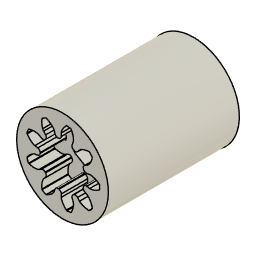
Motor Shaft (Autodesk Fusion 360 design; units mm, degrees)
description: Spur Gear; Module: 1.26; Num Teeth: 9; Pressure Angle: 20.0; Backlash: 0.00 mm
Autodesk Fusion 360 part; units mm, degrees
(part 1 of 2)
sketch "Sketch1" plane through (0, 0, 0) normal (0, 0, 1) x (1, 0, 0) in component "Spur Gear (9 teeth) (1)"
  circle A0 centre (0, 0) radius 4.1072
  circle A1 centre (0, 0) radius 2.5
extrude "Extrude1" add sketch "Sketch1" along normal blind 5 makes body 1 in component "Spur Gear (9 teeth) (1)"
sketch "Sketch2" plane through (0, 0, 0) normal (0, 0, 1) x (1, 0, 0) in component "Spur Gear (9 teeth) (1)"
  spline S0 degree 5 poles (5.2327, -1.0033) (5.2374, -1.0042) (5.2468, -1.0058) (5.2609, -1.0077) (5.2798, -1.0093) (5.3035, -1.0101) (5.3275, -1.0099) (5.3515, -1.0091) (5.3755, -1.008) (5.3996, -1.0067) (5.4238, -1.0051) (5.448, -1.0032) (5.4722, -1.0009) (5.4964, -0.9981) (5.5208, -0.9949) (5.5451, -0.9912) (5.5695, -0.9872) (5.5939, -0.9828) (5.6183, -0.9782) (5.6428, -0.9733) (5.6672, -0.9681) (5.6917, -0.9626) (5.7162, -0.9568) (5.7407, -0.9507) (5.7652, -0.9444) (5.7897, -0.9377) (5.8142, -0.9307) (5.8387, -0.9235) (5.8632, -0.916) (5.8877, -0.9083) (5.9123, -0.9003) (5.9368, -0.892) (5.9613, -0.8835) (5.9858, -0.8747) (6.0103, -0.8657) (6.0347, -0.8565) (6.0592, -0.847) (6.0837, -0.8372) (6.1081, -0.8272) (6.1325, -0.817) (6.1569, -0.8065) (6.1813, -0.7958) (6.2057, -0.7849) (6.23, -0.7738) (6.2543, -0.7624) (6.2786, -0.7508) (6.3029, -0.7389) (6.3271, -0.7269) (6.3513, -0.7146) (6.3755, -0.7021) (6.3997, -0.6894) (6.4238, -0.6765) (6.4479, -0.6633) (6.4719, -0.65) (6.4959, -0.6364) (6.5199, -0.6226) (6.5439, -0.6086) (6.5678, -0.5944) (6.5916, -0.58) (6.6154, -0.5653) (6.6392, -0.5505) (6.663, -0.5355) (6.6866, -0.5202) (6.7103, -0.5048) (6.7339, -0.4892) (6.7574, -0.4733) (6.7809, -0.4573) (6.8044, -0.441) (6.8278, -0.4246) (6.8511, -0.408) (6.8744, -0.3911) (6.893, -0.3775) (6.9069, -0.3672) (6.9162, -0.3603) (6.9208, -0.3568) knots 0 0 0 0 0 0 0.01428571 0.02857143 0.04285714 0.05714286 0.07142857 0.08571429 0.1 0.11428571 0.12857143 0.14285714 0.15714286 0.17142857 0.18571429 0.2 0.21428571 0.22857143 0.24285714 0.25714286 0.27142857 0.28571429 0.3 0.31428571 0.32857143 0.34285714 0.35714286 0.37142857 0.38571429 0.4 0.41428571 0.42857143 0.44285714 0.45714286 0.47142857 0.48571429 0.5 0.51428571 0.52857143 0.54285714 0.55714286 0.57142857 0.58571429 0.6 0.61428571 0.62857143 0.64285714 0.65714286 0.67142857 0.68571429 0.7 0.71428571 0.72857143 0.74285714 0.75714286 0.77142857 0.78571429 0.8 0.81428571 0.82857143 0.84285714 0.85714286 0.87142857 0.88571429 0.9 0.91428571 0.92857143 0.94285714 0.95714286 0.97142857 0.98571429 1 1 1 1 1 1
  spline S1 degree 5 poles (5.2327, 1.0033) (5.2374, 1.0042) (5.2468, 1.0058) (5.2609, 1.0077) (5.2798, 1.0093) (5.3035, 1.0101) (5.3275, 1.0099) (5.3515, 1.0091) (5.3755, 1.008) (5.3996, 1.0067) (5.4238, 1.0051) (5.448, 1.0032) (5.4722, 1.0009) (5.4964, 0.9981) (5.5208, 0.9949) (5.5451, 0.9912) (5.5695, 0.9872) (5.5939, 0.9828) (5.6183, 0.9782) (5.6428, 0.9733) (5.6672, 0.9681) (5.6917, 0.9626) (5.7162, 0.9568) (5.7407, 0.9507) (5.7652, 0.9444) (5.7897, 0.9377) (5.8142, 0.9307) (5.8387, 0.9235) (5.8632, 0.916) (5.8877, 0.9083) (5.9123, 0.9003) (5.9368, 0.892) (5.9613, 0.8835) (5.9858, 0.8747) (6.0103, 0.8657) (6.0347, 0.8565) (6.0592, 0.847) (6.0837, 0.8372) (6.1081, 0.8272) (6.1325, 0.817) (6.1569, 0.8065) (6.1813, 0.7958) (6.2057, 0.7849) (6.23, 0.7738) (6.2543, 0.7624) (6.2786, 0.7508) (6.3029, 0.7389) (6.3271, 0.7269) (6.3513, 0.7146) (6.3755, 0.7021) (6.3997, 0.6894) (6.4238, 0.6765) (6.4479, 0.6633) (6.4719, 0.65) (6.4959, 0.6364) (6.5199, 0.6226) (6.5439, 0.6086) (6.5678, 0.5944) (6.5916, 0.58) (6.6154, 0.5653) (6.6392, 0.5505) (6.663, 0.5355) (6.6866, 0.5202) (6.7103, 0.5048) (6.7339, 0.4892) (6.7574, 0.4733) (6.7809, 0.4573) (6.8044, 0.441) (6.8278, 0.4246) (6.8511, 0.408) (6.8744, 0.3911) (6.893, 0.3775) (6.9069, 0.3672) (6.9162, 0.3603) (6.9208, 0.3568) knots 0 0 0 0 0 0 0.01428571 0.02857143 0.04285714 0.05714286 0.07142857 0.08571429 0.1 0.11428571 0.12857143 0.14285714 0.15714286 0.17142857 0.18571429 0.2 0.21428571 0.22857143 0.24285714 0.25714286 0.27142857 0.28571429 0.3 0.31428571 0.32857143 0.34285714 0.35714286 0.37142857 0.38571429 0.4 0.41428571 0.42857143 0.44285714 0.45714286 0.47142857 0.48571429 0.5 0.51428571 0.52857143 0.54285714 0.55714286 0.57142857 0.58571429 0.6 0.61428571 0.62857143 0.64285714 0.65714286 0.67142857 0.68571429 0.7 0.71428571 0.72857143 0.74285714 0.75714286 0.77142857 0.78571429 0.8 0.81428571 0.82857143 0.84285714 0.85714286 0.87142857 0.88571429 0.9 0.91428571 0.92857143 0.94285714 0.95714286 0.97142857 0.98571429 1 1 1 1 1 1
  arc A0 (6.9208, -0.3568) -> (6.9208, 0.3568) centre (0, 0) ccw
  line L0 (4.0239, -0.7734) -> (5.2327, -1.0033)
  line L1 (4.0239, 0.7734) -> (5.2327, 1.0033)
  line L2 (4.0239, -0.7734) -> (4.0239, 0.7734)
  point P0 (5.3481, -1.0091)
  point P1 (5.4659, -1.0014)
  point P2 (5.5853, -0.9843)
  point P3 (5.7057, -0.9593)
  point P4 (5.8269, -0.9269)
  point P5 (5.9487, -0.8878)
  point P6 (6.0709, -0.8423)
  point P7 (6.1932, -0.7905)
  point P8 (6.3155, -0.7326)
  point P9 (6.4376, -0.6689)
  point P10 (6.5594, -0.5993)
  point P11 (6.6806, -0.5241)
  point P12 (6.8011, -0.4432)
  point P13 (5.3481, 1.0091)
  point P14 (5.4659, 1.0014)
  point P15 (5.5853, 0.9843)
  point P16 (5.7057, 0.9593)
  point P17 (5.8269, 0.9269)
  point P18 (5.9487, 0.8878)
  point P19 (6.0709, 0.8423)
  point P20 (6.1932, 0.7905)
  point P21 (6.3155, 0.7326)
  point P22 (6.4376, 0.6689)
  point P23 (6.5594, 0.5993)
  point P24 (6.6806, 0.5241)
  point P25 (6.8011, 0.4432)
extrude "Extrude2" add sketch "Sketch2" along normal blind 5 bodies 1 in component "Spur Gear (9 teeth) (1)"
fillet "Fillet1" radius 0.7 2 edges at (4.0334, -0.7752, 2.5) (4.0334, 0.7752, 2.5) on bodies 1 in component "Spur Gear (9 teeth) (1)"
pattern_circular "C-Pattern1" count 9 over 360 about axis through (0, 0, 0) along (0, 0, 1) of "Extrude2", "Fillet1" in component "Spur Gear (9 teeth) (1)"
sketch "Sketch3" plane through (0, 0, 0) normal (0, 0, 1) x (1, 0, 0) in component "Spur Gear (9 teeth) (1)"
  circle A0 centre (0, 0) radius 5.67 construction
move_body "Move1" bodies 1 to x (1, 0, 0) y (0, 0, -1) z (0, 1, 0) at (0, -13, 5) in component "Spur Gear (9 teeth) (1)"
sketch "Sketch5" plane through (0, -1, 0) normal (0, -1, 0) x (1, 0, 0)
  circle A0 centre (0, 0) radius 10
  circle A1 centre (0, 5) radius 2.5
  arc A2 (1.6934, 9.443) -> (2.0061, 8.584) centre (2.348, 9.1948) ccw
  line L0 (1.6934, 9.443) -> (1.8967, 9.979)
  spline S0 degree 5 poles (1.8967, 9.979) (1.8984, 9.9835) (1.9016, 9.9924) (1.906, 10.0059) (1.9108, 10.0243) (1.9157, 10.0476) (1.9196, 10.0712) (1.923, 10.0949) (1.9261, 10.1188) (1.929, 10.1428) (1.9316, 10.1668) (1.934, 10.191) (1.9359, 10.2152) (1.9374, 10.2396) (1.9385, 10.2641) (1.9391, 10.2887) (1.9393, 10.3135) (1.9393, 10.3383) (1.9389, 10.3631) (1.9383, 10.388) (1.9375, 10.413) (1.9363, 10.4381) (1.9349, 10.4632) (1.9332, 10.4884) (1.9311, 10.5136) (1.9288, 10.5389) (1.9262, 10.5642) (1.9233, 10.5896) (1.9202, 10.6151) (1.9169, 10.6406) (1.9132, 10.6661) (1.9094, 10.6917) (1.9052, 10.7173) (1.9009, 10.7429) (1.8962, 10.7686) (1.8914, 10.7943) (1.8863, 10.8201) (1.8809, 10.8459) (1.8753, 10.8717) (1.8695, 10.8975) (1.8634, 10.9233) (1.8571, 10.9492) (1.8506, 10.9751) (1.8438, 11.001) (1.8369, 11.0269) (1.8296, 11.0529) (1.8222, 11.0788) (1.8145, 11.1048) (1.8066, 11.1308) (1.7985, 11.1567) (1.7902, 11.1827) (1.7817, 11.2087) (1.7729, 11.2347) (1.7639, 11.2607) (1.7547, 11.2867) (1.7453, 11.3128) (1.7357, 11.3388) (1.7258, 11.3648) (1.7158, 11.3908) (1.7055, 11.4168) (1.695, 11.4428) (1.6844, 11.4687) (1.6735, 11.4947) (1.6624, 11.5207) (1.6511, 11.5466) (1.6395, 11.5726) (1.6278, 11.5985) (1.6159, 11.6244) (1.6038, 11.6503) (1.5914, 11.6762) (1.5789, 11.702) (1.5687, 11.7227) (1.561, 11.7382) (1.5558, 11.7485) (1.5532, 11.7537) knots 0 0 0 0 0 0 0.01428571 0.02857143 0.04285714 0.05714286 0.07142857 0.08571429 0.1 0.11428571 0.12857143 0.14285714 0.15714286 0.17142857 0.18571429 0.2 0.21428571 0.22857143 0.24285714 0.25714286 0.27142857 0.28571429 0.3 0.31428571 0.32857143 0.34285714 0.35714286 0.37142857 0.38571429 0.4 0.41428571 0.42857143 0.44285714 0.45714286 0.47142857 0.48571429 0.5 0.51428571 0.52857143 0.54285714 0.55714286 0.57142857 0.58571429 0.6 0.61428571 0.62857143 0.64285714 0.65714286 0.67142857 0.68571429 0.7 0.71428571 0.72857143 0.74285714 0.75714286 0.77142857 0.78571429 0.8 0.81428571 0.82857143 0.84285714 0.85714286 0.87142857 0.88571429 0.9 0.91428571 0.92857143 0.94285714 0.95714286 0.97142857 0.98571429 1 1 1 1 1 1
  arc A3 (1.5532, 11.7537) -> (0.8504, 11.8776) centre (0, 5) ccw
  spline S1 degree 5 poles (-0.0794, 10.3275) (-0.0795, 10.3322) (-0.0794, 10.3417) (-0.0789, 10.3559) (-0.0772, 10.3748) (-0.0738, 10.3984) (-0.0694, 10.4219) (-0.0645, 10.4454) (-0.0592, 10.4689) (-0.0537, 10.4924) (-0.048, 10.5159) (-0.0419, 10.5394) (-0.0355, 10.5629) (-0.0285, 10.5863) (-0.0211, 10.6097) (-0.0133, 10.633) (-0.0051, 10.6563) (0.0035, 10.6796) (0.0123, 10.7028) (0.0214, 10.726) (0.0307, 10.7492) (0.0404, 10.7724) (0.0503, 10.7955) (0.0606, 10.8185) (0.0711, 10.8416) (0.0819, 10.8645) (0.093, 10.8875) (0.1044, 10.9104) (0.1161, 10.9332) (0.1279, 10.956) (0.1401, 10.9788) (0.1525, 11.0015) (0.1651, 11.0241) (0.178, 11.0467) (0.1911, 11.0693) (0.2045, 11.0918) (0.2181, 11.1142) (0.2319, 11.1366) (0.246, 11.1589) (0.2603, 11.1812) (0.2749, 11.2034) (0.2896, 11.2256) (0.3046, 11.2477) (0.3198, 11.2697) (0.3353, 11.2917) (0.3509, 11.3136) (0.3668, 11.3354) (0.3829, 11.3572) (0.3991, 11.3789) (0.4157, 11.4006) (0.4324, 11.4222) (0.4493, 11.4437) (0.4664, 11.4651) (0.4838, 11.4865) (0.5013, 11.5078) (0.519, 11.529) (0.537, 11.5501) (0.5551, 11.5712) (0.5735, 11.5922) (0.592, 11.6131) (0.6107, 11.634) (0.6297, 11.6547) (0.6488, 11.6754) (0.6681, 11.696) (0.6876, 11.7165) (0.7073, 11.737) (0.7272, 11.7573) (0.7472, 11.7776) (0.7675, 11.7978) (0.7879, 11.8179) (0.8086, 11.8379) (0.8252, 11.8538) (0.8378, 11.8657) (0.8462, 11.8737) (0.8504, 11.8776) knots 0 0 0 0 0 0 0.01428571 0.02857143 0.04285714 0.05714286 0.07142857 0.08571429 0.1 0.11428571 0.12857143 0.14285714 0.15714286 0.17142857 0.18571429 0.2 0.21428571 0.22857143 0.24285714 0.25714286 0.27142857 0.28571429 0.3 0.31428571 0.32857143 0.34285714 0.35714286 0.37142857 0.38571429 0.4 0.41428571 0.42857143 0.44285714 0.45714286 0.47142857 0.48571429 0.5 0.51428571 0.52857143 0.54285714 0.55714286 0.57142857 0.58571429 0.6 0.61428571 0.62857143 0.64285714 0.65714286 0.67142857 0.68571429 0.7 0.71428571 0.72857143 0.74285714 0.75714286 0.77142857 0.78571429 0.8 0.81428571 0.82857143 0.84285714 0.85714286 0.87142857 0.88571429 0.9 0.91428571 0.92857143 0.94285714 0.95714286 0.97142857 0.98571429 1 1 1 1 1 1
  line L1 (-0.0794, 10.3275) -> (-0.0717, 9.7542)
  arc A4 (-0.6593, 9.0539) -> (-0.0717, 9.7542) centre (-0.7717, 9.7449) ccw
  arc A5 (-0.6593, 9.0539) -> (-0.767, 9.0349) centre (0, 5) ccw
  arc A6 (-1.5586, 9.4921) -> (-0.767, 9.0349) centre (-0.8977, 9.7226) ccw
  line L2 (-1.5586, 9.4921) -> (-1.7475, 10.0333)
  spline S2 degree 5 poles (-1.7475, 10.0333) (-1.749, 10.0378) (-1.7523, 10.0467) (-1.7577, 10.0599) (-1.7658, 10.0771) (-1.777, 10.098) (-1.7892, 10.1187) (-1.8018, 10.1391) (-1.8148, 10.1593) (-1.828, 10.1795) (-1.8415, 10.1997) (-1.8552, 10.2197) (-1.8693, 10.2395) (-1.8838, 10.2591) (-1.8988, 10.2786) (-1.9141, 10.2978) (-1.9298, 10.3169) (-1.9458, 10.3359) (-1.962, 10.3547) (-1.9785, 10.3734) (-1.9952, 10.392) (-2.0122, 10.4104) (-2.0294, 10.4288) (-2.047, 10.4469) (-2.0647, 10.465) (-2.0828, 10.4828) (-2.1011, 10.5006) (-2.1196, 10.5182) (-2.1383, 10.5357) (-2.1573, 10.5531) (-2.1765, 10.5703) (-2.1959, 10.5874) (-2.2155, 10.6044) (-2.2353, 10.6212) (-2.2554, 10.6379) (-2.2757, 10.6545) (-2.2961, 10.6709) (-2.3168, 10.6872) (-2.3377, 10.7034) (-2.3587, 10.7194) (-2.38, 10.7353) (-2.4014, 10.7511) (-2.4231, 10.7667) (-2.4449, 10.7822) (-2.4669, 10.7976) (-2.4891, 10.8128) (-2.5115, 10.8279) (-2.5341, 10.8429) (-2.5568, 10.8577) (-2.5797, 10.8724) (-2.6028, 10.887) (-2.6261, 10.9014) (-2.6495, 10.9157) (-2.6731, 10.9298) (-2.6969, 10.9438) (-2.7208, 10.9577) (-2.7449, 10.9714) (-2.7691, 10.985) (-2.7935, 10.9985) (-2.8181, 11.0118) (-2.8429, 11.025) (-2.8677, 11.038) (-2.8928, 11.0509) (-2.918, 11.0637) (-2.9433, 11.0763) (-2.9688, 11.0888) (-2.9945, 11.1011) (-3.0202, 11.1133) (-3.0462, 11.1253) (-3.0723, 11.1372) (-3.0985, 11.149) (-3.1196, 11.1583) (-3.1355, 11.1652) (-3.1461, 11.1697) (-3.1514, 11.172) knots 0 0 0 0 0 0 0.01428571 0.02857143 0.04285714 0.05714286 0.07142857 0.08571429 0.1 0.11428571 0.12857143 0.14285714 0.15714286 0.17142857 0.18571429 0.2 0.21428571 0.22857143 0.24285714 0.25714286 0.27142857 0.28571429 0.3 0.31428571 0.32857143 0.34285714 0.35714286 0.37142857 0.38571429 0.4 0.41428571 0.42857143 0.44285714 0.45714286 0.47142857 0.48571429 0.5 0.51428571 0.52857143 0.54285714 0.55714286 0.57142857 0.58571429 0.6 0.61428571 0.62857143 0.64285714 0.65714286 0.67142857 0.68571429 0.7 0.71428571 0.72857143 0.74285714 0.75714286 0.77142857 0.78571429 0.8 0.81428571 0.82857143 0.84285714 0.85714286 0.87142857 0.88571429 0.9 0.91428571 0.92857143 0.94285714 0.95714286 0.97142857 0.98571429 1 1 1 1 1 1
  arc A7 (-3.1514, 11.172) -> (-3.7694, 10.8152) centre (0, 5) ccw
  spline S3 degree 5 poles (-3.4853, 9.03) (-3.4884, 9.0336) (-3.4944, 9.0409) (-3.5031, 9.0522) (-3.514, 9.0677) (-3.5265, 9.088) (-3.5383, 9.1088) (-3.5496, 9.13) (-3.5607, 9.1514) (-3.5716, 9.1729) (-3.5823, 9.1946) (-3.5928, 9.2165) (-3.6029, 9.2386) (-3.6126, 9.261) (-3.622, 9.2837) (-3.631, 9.3066) (-3.6397, 9.3297) (-3.6481, 9.353) (-3.6563, 9.3765) (-3.6643, 9.4001) (-3.672, 9.4239) (-3.6795, 9.4478) (-3.6867, 9.4719) (-3.6937, 9.4962) (-3.7004, 9.5206) (-3.7069, 9.5452) (-3.7131, 9.5699) (-3.7191, 9.5947) (-3.7249, 9.6197) (-3.7305, 9.6448) (-3.7358, 9.67) (-3.7409, 9.6954) (-3.7458, 9.7209) (-3.7504, 9.7465) (-3.7549, 9.7722) (-3.7591, 9.798) (-3.7631, 9.8239) (-3.7669, 9.85) (-3.7704, 9.8762) (-3.7738, 9.9024) (-3.7769, 9.9288) (-3.7799, 9.9552) (-3.7826, 9.9818) (-3.7851, 10.0085) (-3.7874, 10.0352) (-3.7895, 10.0621) (-3.7914, 10.089) (-3.7931, 10.116) (-3.7945, 10.1431) (-3.7958, 10.1703) (-3.7969, 10.1976) (-3.7977, 10.2249) (-3.7984, 10.2524) (-3.7988, 10.2799) (-3.7991, 10.3075) (-3.7991, 10.3351) (-3.799, 10.3629) (-3.7986, 10.3907) (-3.7981, 10.4185) (-3.7973, 10.4465) (-3.7964, 10.4745) (-3.7952, 10.5026) (-3.7939, 10.5307) (-3.7923, 10.5589) (-3.7906, 10.5871) (-3.7886, 10.6155) (-3.7865, 10.6438) (-3.7841, 10.6723) (-3.7816, 10.7007) (-3.7789, 10.7293) (-3.7759, 10.7578) (-3.7734, 10.7808) (-3.7715, 10.798) (-3.7701, 10.8094) (-3.7694, 10.8152) knots 0 0 0 0 0 0 0.01428571 0.02857143 0.04285714 0.05714286 0.07142857 0.08571429 0.1 0.11428571 0.12857143 0.14285714 0.15714286 0.17142857 0.18571429 0.2 0.21428571 0.22857143 0.24285714 0.25714286 0.27142857 0.28571429 0.3 0.31428571 0.32857143 0.34285714 0.35714286 0.37142857 0.38571429 0.4 0.41428571 0.42857143 0.44285714 0.45714286 0.47142857 0.48571429 0.5 0.51428571 0.52857143 0.54285714 0.55714286 0.57142857 0.58571429 0.6 0.61428571 0.62857143 0.64285714 0.65714286 0.67142857 0.68571429 0.7 0.71428571 0.72857143 0.74285714 0.75714286 0.77142857 0.78571429 0.8 0.81428571 0.82857143 0.84285714 0.85714286 0.87142857 0.88571429 0.9 0.91428571 0.92857143 0.94285714 0.95714286 0.97142857 0.98571429 1 1 1 1 1 1
  line L3 (-3.4853, 9.03) -> (-3.1109, 8.5959)
  arc A8 (-3.1109, 7.6817) -> (-3.1109, 8.5959) centre (-3.6411, 8.1388) ccw
  arc A9 (-3.1109, 7.6817) -> (-3.1812, 7.5979) centre (0, 5) ccw
  arc A10 (-4.0814, 7.4392) -> (-3.1812, 7.5979) centre (-3.7233, 8.0407) ccw
  line L4 (-4.0814, 7.4392) -> (-4.574, 7.7325)
  spline S4 degree 5 poles (-4.574, 7.7325) (-4.5781, 7.7349) (-4.5863, 7.7396) (-4.5989, 7.7463) (-4.6161, 7.7543) (-4.6382, 7.7631) (-4.6608, 7.7711) (-4.6836, 7.7786) (-4.7066, 7.7857) (-4.7297, 7.7927) (-4.7529, 7.7995) (-4.7763, 7.806) (-4.7998, 7.8121) (-4.8236, 7.8178) (-4.8475, 7.8231) (-4.8717, 7.828) (-4.896, 7.8325) (-4.9204, 7.8368) (-4.9449, 7.8408) (-4.9696, 7.8445) (-4.9943, 7.848) (-5.0192, 7.8512) (-5.0442, 7.8542) (-5.0693, 7.8568) (-5.0945, 7.8592) (-5.1198, 7.8613) (-5.1452, 7.8632) (-5.1707, 7.8648) (-5.1963, 7.8661) (-5.222, 7.8672) (-5.2478, 7.8681) (-5.2737, 7.8687) (-5.2996, 7.8691) (-5.3256, 7.8692) (-5.3517, 7.8691) (-5.3779, 7.8688) (-5.4041, 7.8682) (-5.4304, 7.8674) (-5.4568, 7.8664) (-5.4832, 7.8652) (-5.5098, 7.8637) (-5.5363, 7.862) (-5.563, 7.86) (-5.5896, 7.8579) (-5.6164, 7.8555) (-5.6432, 7.8529) (-5.67, 7.8501) (-5.6969, 7.8471) (-5.7239, 7.8438) (-5.7509, 7.8403) (-5.7779, 7.8366) (-5.805, 7.8327) (-5.8322, 7.8286) (-5.8593, 7.8243) (-5.8865, 7.8197) (-5.9138, 7.815) (-5.9411, 7.81) (-5.9684, 7.8048) (-5.9957, 7.7995) (-6.0231, 7.7939) (-6.0505, 7.7881) (-6.078, 7.7821) (-6.1055, 7.7758) (-6.133, 7.7694) (-6.1605, 7.7628) (-6.188, 7.7559) (-6.2156, 7.7489) (-6.2432, 7.7417) (-6.2708, 7.7342) (-6.2984, 7.7266) (-6.3261, 7.7187) (-6.3482, 7.7123) (-6.3648, 7.7073) (-6.3759, 7.704) (-6.3814, 7.7024) knots 0 0 0 0 0 0 0.01428571 0.02857143 0.04285714 0.05714286 0.07142857 0.08571429 0.1 0.11428571 0.12857143 0.14285714 0.15714286 0.17142857 0.18571429 0.2 0.21428571 0.22857143 0.24285714 0.25714286 0.27142857 0.28571429 0.3 0.31428571 0.32857143 0.34285714 0.35714286 0.37142857 0.38571429 0.4 0.41428571 0.42857143 0.44285714 0.45714286 0.47142857 0.48571429 0.5 0.51428571 0.52857143 0.54285714 0.55714286 0.57142857 0.58571429 0.6 0.61428571 0.62857143 0.64285714 0.65714286 0.67142857 0.68571429 0.7 0.71428571 0.72857143 0.74285714 0.75714286 0.77142857 0.78571429 0.8 0.81428571 0.82857143 0.84285714 0.85714286 0.87142857 0.88571429 0.9 0.91428571 0.92857143 0.94285714 0.95714286 0.97142857 0.98571429 1 1 1 1 1 1
  arc A11 (-6.3814, 7.7024) -> (-6.6255, 7.0318) centre (0, 5) ccw
  spline S5 degree 5 poles (-5.2603, 5.8469) (-5.265, 5.8477) (-5.2743, 5.8494) (-5.2882, 5.8524) (-5.3066, 5.8573) (-5.3292, 5.8648) (-5.3516, 5.8731) (-5.3739, 5.8821) (-5.3961, 5.8913) (-5.4183, 5.9008) (-5.4404, 5.9106) (-5.4625, 5.9206) (-5.4845, 5.9311) (-5.5064, 5.942) (-5.5281, 5.9533) (-5.5497, 5.9651) (-5.5713, 5.9772) (-5.5927, 5.9897) (-5.6141, 6.0024) (-5.6353, 6.0154) (-5.6565, 6.0286) (-5.6777, 6.0421) (-5.6987, 6.0559) (-5.7196, 6.07) (-5.7405, 6.0844) (-5.7612, 6.0991) (-5.7819, 6.114) (-5.8024, 6.1292) (-5.8229, 6.1446) (-5.8433, 6.1602) (-5.8636, 6.1761) (-5.8838, 6.1923) (-5.9039, 6.2087) (-5.924, 6.2253) (-5.9439, 6.2421) (-5.9637, 6.2592) (-5.9835, 6.2765) (-6.0031, 6.294) (-6.0227, 6.3118) (-6.0421, 6.3297) (-6.0615, 6.3479) (-6.0807, 6.3663) (-6.0999, 6.3849) (-6.1189, 6.4037) (-6.1379, 6.4227) (-6.1567, 6.4419) (-6.1755, 6.4613) (-6.1942, 6.481) (-6.2127, 6.5008) (-6.2312, 6.5208) (-6.2495, 6.541) (-6.2678, 6.5614) (-6.2859, 6.582) (-6.3039, 6.6028) (-6.3218, 6.6237) (-6.3397, 6.6449) (-6.3574, 6.6662) (-6.375, 6.6878) (-6.3925, 6.7095) (-6.4098, 6.7314) (-6.4271, 6.7534) (-6.4443, 6.7757) (-6.4613, 6.7981) (-6.4783, 6.8207) (-6.4951, 6.8435) (-6.5118, 6.8664) (-6.5284, 6.8895) (-6.5449, 6.9128) (-6.5612, 6.9363) (-6.5775, 6.9599) (-6.5936, 6.9837) (-6.6064, 7.0028) (-6.616, 7.0173) (-6.6223, 7.0269) (-6.6255, 7.0318) knots 0 0 0 0 0 0 0.01428571 0.02857143 0.04285714 0.05714286 0.07142857 0.08571429 0.1 0.11428571 0.12857143 0.14285714 0.15714286 0.17142857 0.18571429 0.2 0.21428571 0.22857143 0.24285714 0.25714286 0.27142857 0.28571429 0.3 0.31428571 0.32857143 0.34285714 0.35714286 0.37142857 0.38571429 0.4 0.41428571 0.42857143 0.44285714 0.45714286 0.47142857 0.48571429 0.5 0.51428571 0.52857143 0.54285714 0.55714286 0.57142857 0.58571429 0.6 0.61428571 0.62857143 0.64285714 0.65714286 0.67142857 0.68571429 0.7 0.71428571 0.72857143 0.74285714 0.75714286 0.77142857 0.78571429 0.8 0.81428571 0.82857143 0.84285714 0.85714286 0.87142857 0.88571429 0.9 0.91428571 0.92857143 0.94285714 0.95714286 0.97142857 0.98571429 1 1 1 1 1 1
  line L5 (-5.2603, 5.8469) -> (-4.6945, 5.7549)
  arc A12 (-4.1068, 5.0547) -> (-4.6945, 5.7549) centre (-4.8068, 5.064) ccw
  arc A13 (-4.1068, 5.0547) -> (-4.1068, 4.9453) centre (0, 5) ccw
  arc A14 (-4.6945, 4.2451) -> (-4.1068, 4.9453) centre (-4.8068, 4.936) ccw
  line L6 (-4.6945, 4.2451) -> (-5.2603, 4.1531)
  spline S6 degree 5 poles (-5.2603, 4.1531) (-5.265, 4.1523) (-5.2743, 4.1506) (-5.2882, 4.1476) (-5.3066, 4.1427) (-5.3292, 4.1352) (-5.3516, 4.1269) (-5.3739, 4.1179) (-5.3961, 4.1087) (-5.4183, 4.0992) (-5.4404, 4.0894) (-5.4625, 4.0794) (-5.4845, 4.0689) (-5.5064, 4.058) (-5.5281, 4.0467) (-5.5497, 4.0349) (-5.5713, 4.0228) (-5.5927, 4.0103) (-5.6141, 3.9976) (-5.6353, 3.9846) (-5.6565, 3.9714) (-5.6777, 3.9579) (-5.6987, 3.9441) (-5.7196, 3.93) (-5.7405, 3.9156) (-5.7612, 3.9009) (-5.7819, 3.886) (-5.8024, 3.8708) (-5.8229, 3.8554) (-5.8433, 3.8398) (-5.8636, 3.8239) (-5.8838, 3.8077) (-5.9039, 3.7913) (-5.924, 3.7747) (-5.9439, 3.7579) (-5.9637, 3.7408) (-5.9835, 3.7235) (-6.0031, 3.706) (-6.0227, 3.6882) (-6.0421, 3.6703) (-6.0615, 3.6521) (-6.0807, 3.6337) (-6.0999, 3.6151) (-6.1189, 3.5963) (-6.1379, 3.5773) (-6.1567, 3.5581) (-6.1755, 3.5387) (-6.1942, 3.519) (-6.2127, 3.4992) (-6.2312, 3.4792) (-6.2495, 3.459) (-6.2678, 3.4386) (-6.2859, 3.418) (-6.3039, 3.3972) (-6.3218, 3.3763) (-6.3397, 3.3551) (-6.3574, 3.3338) (-6.375, 3.3122) (-6.3925, 3.2905) (-6.4098, 3.2686) (-6.4271, 3.2466) (-6.4443, 3.2243) (-6.4613, 3.2019) (-6.4783, 3.1793) (-6.4951, 3.1565) (-6.5118, 3.1336) (-6.5284, 3.1105) (-6.5449, 3.0872) (-6.5612, 3.0637) (-6.5775, 3.0401) (-6.5936, 3.0163) (-6.6064, 2.9972) (-6.616, 2.9827) (-6.6223, 2.9731) (-6.6255, 2.9682) knots 0 0 0 0 0 0 0.01428571 0.02857143 0.04285714 0.05714286 0.07142857 0.08571429 0.1 0.11428571 0.12857143 0.14285714 0.15714286 0.17142857 0.18571429 0.2 0.21428571 0.22857143 0.24285714 0.25714286 0.27142857 0.28571429 0.3 0.31428571 0.32857143 0.34285714 0.35714286 0.37142857 0.38571429 0.4 0.41428571 0.42857143 0.44285714 0.45714286 0.47142857 0.48571429 0.5 0.51428571 0.52857143 0.54285714 0.55714286 0.57142857 0.58571429 0.6 0.61428571 0.62857143 0.64285714 0.65714286 0.67142857 0.68571429 0.7 0.71428571 0.72857143 0.74285714 0.75714286 0.77142857 0.78571429 0.8 0.81428571 0.82857143 0.84285714 0.85714286 0.87142857 0.88571429 0.9 0.91428571 0.92857143 0.94285714 0.95714286 0.97142857 0.98571429 1 1 1 1 1 1
  arc A15 (-6.6255, 2.9682) -> (-6.3814, 2.2976) centre (0, 5) ccw
  spline S7 degree 5 poles (-4.574, 2.2675) (-4.5781, 2.2651) (-4.5863, 2.2604) (-4.5989, 2.2537) (-4.6161, 2.2457) (-4.6382, 2.2369) (-4.6608, 2.2289) (-4.6836, 2.2214) (-4.7066, 2.2143) (-4.7297, 2.2073) (-4.7529, 2.2005) (-4.7763, 2.194) (-4.7998, 2.1879) (-4.8236, 2.1822) (-4.8475, 2.1769) (-4.8717, 2.172) (-4.896, 2.1675) (-4.9204, 2.1632) (-4.9449, 2.1592) (-4.9696, 2.1555) (-4.9943, 2.152) (-5.0192, 2.1488) (-5.0442, 2.1458) (-5.0693, 2.1432) (-5.0945, 2.1408) (-5.1198, 2.1387) (-5.1452, 2.1368) (-5.1707, 2.1352) (-5.1963, 2.1339) (-5.222, 2.1328) (-5.2478, 2.1319) (-5.2737, 2.1313) (-5.2996, 2.1309) (-5.3256, 2.1308) (-5.3517, 2.1309) (-5.3779, 2.1312) (-5.4041, 2.1318) (-5.4304, 2.1326) (-5.4568, 2.1336) (-5.4832, 2.1348) (-5.5098, 2.1363) (-5.5363, 2.138) (-5.563, 2.14) (-5.5896, 2.1421) (-5.6164, 2.1445) (-5.6432, 2.1471) (-5.67, 2.1499) (-5.6969, 2.1529) (-5.7239, 2.1562) (-5.7509, 2.1597) (-5.7779, 2.1634) (-5.805, 2.1673) (-5.8322, 2.1714) (-5.8593, 2.1757) (-5.8865, 2.1803) (-5.9138, 2.185) (-5.9411, 2.19) (-5.9684, 2.1952) (-5.9957, 2.2005) (-6.0231, 2.2061) (-6.0505, 2.2119) (-6.078, 2.2179) (-6.1055, 2.2242) (-6.133, 2.2306) (-6.1605, 2.2372) (-6.188, 2.2441) (-6.2156, 2.2511) (-6.2432, 2.2583) (-6.2708, 2.2658) (-6.2984, 2.2734) (-6.3261, 2.2813) (-6.3482, 2.2877) (-6.3648, 2.2927) (-6.3759, 2.296) (-6.3814, 2.2976) knots 0 0 0 0 0 0 0.01428571 0.02857143 0.04285714 0.05714286 0.07142857 0.08571429 0.1 0.11428571 0.12857143 0.14285714 0.15714286 0.17142857 0.18571429 0.2 0.21428571 0.22857143 0.24285714 0.25714286 0.27142857 0.28571429 0.3 0.31428571 0.32857143 0.34285714 0.35714286 0.37142857 0.38571429 0.4 0.41428571 0.42857143 0.44285714 0.45714286 0.47142857 0.48571429 0.5 0.51428571 0.52857143 0.54285714 0.55714286 0.57142857 0.58571429 0.6 0.61428571 0.62857143 0.64285714 0.65714286 0.67142857 0.68571429 0.7 0.71428571 0.72857143 0.74285714 0.75714286 0.77142857 0.78571429 0.8 0.81428571 0.82857143 0.84285714 0.85714286 0.87142857 0.88571429 0.9 0.91428571 0.92857143 0.94285714 0.95714286 0.97142857 0.98571429 1 1 1 1 1 1
  line L7 (-4.574, 2.2675) -> (-4.0814, 2.5608)
  arc A16 (-3.1812, 2.4021) -> (-4.0814, 2.5608) centre (-3.7233, 1.9593) ccw
  arc A17 (-3.1812, 2.4021) -> (-3.1109, 2.3183) centre (0, 5) ccw
  arc A18 (-3.1109, 1.4041) -> (-3.1109, 2.3183) centre (-3.6411, 1.8612) ccw
  line L8 (-3.1109, 1.4041) -> (-3.4853, 0.97)
  spline S8 degree 5 poles (-3.4853, 0.97) (-3.4884, 0.9664) (-3.4944, 0.9591) (-3.5031, 0.9478) (-3.514, 0.9323) (-3.5265, 0.912) (-3.5383, 0.8912) (-3.5496, 0.87) (-3.5607, 0.8486) (-3.5716, 0.8271) (-3.5823, 0.8054) (-3.5928, 0.7835) (-3.6029, 0.7614) (-3.6126, 0.739) (-3.622, 0.7163) (-3.631, 0.6934) (-3.6397, 0.6703) (-3.6481, 0.647) (-3.6563, 0.6235) (-3.6643, 0.5999) (-3.672, 0.5761) (-3.6795, 0.5522) (-3.6867, 0.5281) (-3.6937, 0.5038) (-3.7004, 0.4794) (-3.7069, 0.4548) (-3.7131, 0.4301) (-3.7191, 0.4053) (-3.7249, 0.3803) (-3.7305, 0.3552) (-3.7358, 0.33) (-3.7409, 0.3046) (-3.7458, 0.2791) (-3.7504, 0.2535) (-3.7549, 0.2278) (-3.7591, 0.202) (-3.7631, 0.1761) (-3.7669, 0.15) (-3.7704, 0.1238) (-3.7738, 0.0976) (-3.7769, 0.0712) (-3.7799, 0.0448) (-3.7826, 0.0182) (-3.7851, -0.0085) (-3.7874, -0.0352) (-3.7895, -0.0621) (-3.7914, -0.089) (-3.7931, -0.116) (-3.7945, -0.1431) (-3.7958, -0.1703) (-3.7969, -0.1976) (-3.7977, -0.2249) (-3.7984, -0.2524) (-3.7988, -0.2799) (-3.7991, -0.3075) (-3.7991, -0.3351) (-3.799, -0.3629) (-3.7986, -0.3907) (-3.7981, -0.4185) (-3.7973, -0.4465) (-3.7964, -0.4745) (-3.7952, -0.5026) (-3.7939, -0.5307) (-3.7923, -0.5589) (-3.7906, -0.5871) (-3.7886, -0.6155) (-3.7865, -0.6438) (-3.7841, -0.6723) (-3.7816, -0.7007) (-3.7789, -0.7293) (-3.7759, -0.7578) (-3.7734, -0.7808) (-3.7715, -0.798) (-3.7701, -0.8094) (-3.7694, -0.8152) knots 0 0 0 0 0 0 0.01428571 0.02857143 0.04285714 0.05714286 0.07142857 0.08571429 0.1 0.11428571 0.12857143 0.14285714 0.15714286 0.17142857 0.18571429 0.2 0.21428571 0.22857143 0.24285714 0.25714286 0.27142857 0.28571429 0.3 0.31428571 0.32857143 0.34285714 0.35714286 0.37142857 0.38571429 0.4 0.41428571 0.42857143 0.44285714 0.45714286 0.47142857 0.48571429 0.5 0.51428571 0.52857143 0.54285714 0.55714286 0.57142857 0.58571429 0.6 0.61428571 0.62857143 0.64285714 0.65714286 0.67142857 0.68571429 0.7 0.71428571 0.72857143 0.74285714 0.75714286 0.77142857 0.78571429 0.8 0.81428571 0.82857143 0.84285714 0.85714286 0.87142857 0.88571429 0.9 0.91428571 0.92857143 0.94285714 0.95714286 0.97142857 0.98571429 1 1 1 1 1 1
  arc A19 (-3.7694, -0.8152) -> (-3.1514, -1.172) centre (0, 5) ccw
  spline S9 degree 5 poles (-1.7475, -0.0333) (-1.749, -0.0378) (-1.7523, -0.0467) (-1.7577, -0.0599) (-1.7658, -0.0771) (-1.777, -0.098) (-1.7892, -0.1187) (-1.8018, -0.1391) (-1.8148, -0.1593) (-1.828, -0.1795) (-1.8415, -0.1997) (-1.8552, -0.2197) (-1.8693, -0.2395) (-1.8838, -0.2591) (-1.8988, -0.2786) (-1.9141, -0.2978) (-1.9298, -0.3169) (-1.9458, -0.3359) (-1.962, -0.3547) (-1.9785, -0.3734) (-1.9952, -0.392) (-2.0122, -0.4104) (-2.0294, -0.4288) (-2.047, -0.4469) (-2.0647, -0.465) (-2.0828, -0.4828) (-2.1011, -0.5006) (-2.1196, -0.5182) (-2.1383, -0.5357) (-2.1573, -0.5531) (-2.1765, -0.5703) (-2.1959, -0.5874) (-2.2155, -0.6044) (-2.2353, -0.6212) (-2.2554, -0.6379) (-2.2757, -0.6545) (-2.2961, -0.6709) (-2.3168, -0.6872) (-2.3377, -0.7034) (-2.3587, -0.7194) (-2.38, -0.7353) (-2.4014, -0.7511) (-2.4231, -0.7667) (-2.4449, -0.7822) (-2.4669, -0.7976) (-2.4891, -0.8128) (-2.5115, -0.8279) (-2.5341, -0.8429) (-2.5568, -0.8577) (-2.5797, -0.8724) (-2.6028, -0.887) (-2.6261, -0.9014) (-2.6495, -0.9157) (-2.6731, -0.9298) (-2.6969, -0.9438) (-2.7208, -0.9577) (-2.7449, -0.9714) (-2.7691, -0.985) (-2.7935, -0.9985) (-2.8181, -1.0118) (-2.8429, -1.025) (-2.8677, -1.038) (-2.8928, -1.0509) (-2.918, -1.0637) (-2.9433, -1.0763) (-2.9688, -1.0888) (-2.9945, -1.1011) (-3.0202, -1.1133) (-3.0462, -1.1253) (-3.0723, -1.1372) (-3.0985, -1.149) (-3.1196, -1.1583) (-3.1355, -1.1652) (-3.1461, -1.1697) (-3.1514, -1.172) knots 0 0 0 0 0 0 0.01428571 0.02857143 0.04285714 0.05714286 0.07142857 0.08571429 0.1 0.11428571 0.12857143 0.14285714 0.15714286 0.17142857 0.18571429 0.2 0.21428571 0.22857143 0.24285714 0.25714286 0.27142857 0.28571429 0.3 0.31428571 0.32857143 0.34285714 0.35714286 0.37142857 0.38571429 0.4 0.41428571 0.42857143 0.44285714 0.45714286 0.47142857 0.48571429 0.5 0.51428571 0.52857143 0.54285714 0.55714286 0.57142857 0.58571429 0.6 0.61428571 0.62857143 0.64285714 0.65714286 0.67142857 0.68571429 0.7 0.71428571 0.72857143 0.74285714 0.75714286 0.77142857 0.78571429 0.8 0.81428571 0.82857143 0.84285714 0.85714286 0.87142857 0.88571429 0.9 0.91428571 0.92857143 0.94285714 0.95714286 0.97142857 0.98571429 1 1 1 1 1 1
  line L9 (-1.7475, -0.0333) -> (-1.5586, 0.5079)
  arc A20 (-0.767, 0.9651) -> (-1.5586, 0.5079) centre (-0.8977, 0.2774) ccw
  arc A21 (-0.767, 0.9651) -> (-0.6593, 0.9461) centre (0, 5) ccw
  arc A22 (-0.0717, 0.2458) -> (-0.6593, 0.9461) centre (-0.7717, 0.2551) ccw
  line L10 (-0.0717, 0.2458) -> (-0.0794, -0.3275)
  spline S10 degree 5 poles (-0.0794, -0.3275) (-0.0795, -0.3322) (-0.0794, -0.3417) (-0.0789, -0.3559) (-0.0772, -0.3748) (-0.0738, -0.3984) (-0.0694, -0.4219) (-0.0645, -0.4454) (-0.0592, -0.4689) (-0.0537, -0.4924) (-0.048, -0.5159) (-0.0419, -0.5394) (-0.0355, -0.5629) (-0.0285, -0.5863) (-0.0211, -0.6097) (-0.0133, -0.633) (-0.0051, -0.6563) (0.0035, -0.6796) (0.0123, -0.7028) (0.0214, -0.726) (0.0307, -0.7492) (0.0404, -0.7724) (0.0503, -0.7955) (0.0606, -0.8185) (0.0711, -0.8416) (0.0819, -0.8645) (0.093, -0.8875) (0.1044, -0.9104) (0.1161, -0.9332) (0.1279, -0.956) (0.1401, -0.9788) (0.1525, -1.0015) (0.1651, -1.0241) (0.178, -1.0467) (0.1911, -1.0693) (0.2045, -1.0918) (0.2181, -1.1142) (0.2319, -1.1366) (0.246, -1.1589) (0.2603, -1.1812) (0.2749, -1.2034) (0.2896, -1.2256) (0.3046, -1.2477) (0.3198, -1.2697) (0.3353, -1.2917) (0.3509, -1.3136) (0.3668, -1.3354) (0.3829, -1.3572) (0.3991, -1.3789) (0.4157, -1.4006) (0.4324, -1.4222) (0.4493, -1.4437) (0.4664, -1.4651) (0.4838, -1.4865) (0.5013, -1.5078) (0.519, -1.529) (0.537, -1.5501) (0.5551, -1.5712) (0.5735, -1.5922) (0.592, -1.6131) (0.6107, -1.634) (0.6297, -1.6547) (0.6488, -1.6754) (0.6681, -1.696) (0.6876, -1.7165) (0.7073, -1.737) (0.7272, -1.7573) (0.7472, -1.7776) (0.7675, -1.7978) (0.7879, -1.8179) (0.8086, -1.8379) (0.8252, -1.8538) (0.8378, -1.8657) (0.8462, -1.8737) (0.8504, -1.8776) knots 0 0 0 0 0 0 0.01428571 0.02857143 0.04285714 0.05714286 0.07142857 0.08571429 0.1 0.11428571 0.12857143 0.14285714 0.15714286 0.17142857 0.18571429 0.2 0.21428571 0.22857143 0.24285714 0.25714286 0.27142857 0.28571429 0.3 0.31428571 0.32857143 0.34285714 0.35714286 0.37142857 0.38571429 0.4 0.41428571 0.42857143 0.44285714 0.45714286 0.47142857 0.48571429 0.5 0.51428571 0.52857143 0.54285714 0.55714286 0.57142857 0.58571429 0.6 0.61428571 0.62857143 0.64285714 0.65714286 0.67142857 0.68571429 0.7 0.71428571 0.72857143 0.74285714 0.75714286 0.77142857 0.78571429 0.8 0.81428571 0.82857143 0.84285714 0.85714286 0.87142857 0.88571429 0.9 0.91428571 0.92857143 0.94285714 0.95714286 0.97142857 0.98571429 1 1 1 1 1 1
  arc A23 (0.8504, -1.8776) -> (1.5532, -1.7537) centre (0, 5) ccw
  spline S11 degree 5 poles (1.8967, 0.021) (1.8984, 0.0165) (1.9016, 0.0076) (1.906, -0.0059) (1.9108, -0.0243) (1.9157, -0.0476) (1.9196, -0.0712) (1.923, -0.0949) (1.9261, -0.1188) (1.929, -0.1428) (1.9316, -0.1668) (1.934, -0.191) (1.9359, -0.2152) (1.9374, -0.2396) (1.9385, -0.2641) (1.9391, -0.2887) (1.9393, -0.3135) (1.9393, -0.3383) (1.9389, -0.3631) (1.9383, -0.388) (1.9375, -0.413) (1.9363, -0.4381) (1.9349, -0.4632) (1.9332, -0.4884) (1.9311, -0.5136) (1.9288, -0.5389) (1.9262, -0.5642) (1.9233, -0.5896) (1.9202, -0.6151) (1.9169, -0.6406) (1.9132, -0.6661) (1.9094, -0.6917) (1.9052, -0.7173) (1.9009, -0.7429) (1.8962, -0.7686) (1.8914, -0.7943) (1.8863, -0.8201) (1.8809, -0.8459) (1.8753, -0.8717) (1.8695, -0.8975) (1.8634, -0.9233) (1.8571, -0.9492) (1.8506, -0.9751) (1.8438, -1.001) (1.8369, -1.0269) (1.8296, -1.0529) (1.8222, -1.0788) (1.8145, -1.1048) (1.8066, -1.1308) (1.7985, -1.1567) (1.7902, -1.1827) (1.7817, -1.2087) (1.7729, -1.2347) (1.7639, -1.2607) (1.7547, -1.2867) (1.7453, -1.3128) (1.7357, -1.3388) (1.7258, -1.3648) (1.7158, -1.3908) (1.7055, -1.4168) (1.695, -1.4428) (1.6844, -1.4687) (1.6735, -1.4947) (1.6624, -1.5207) (1.6511, -1.5466) (1.6395, -1.5726) (1.6278, -1.5985) (1.6159, -1.6244) (1.6038, -1.6503) (1.5914, -1.6762) (1.5789, -1.702) (1.5687, -1.7227) (1.561, -1.7382) (1.5558, -1.7485) (1.5532, -1.7537) knots 0 0 0 0 0 0 0.01428571 0.02857143 0.04285714 0.05714286 0.07142857 0.08571429 0.1 0.11428571 0.12857143 0.14285714 0.15714286 0.17142857 0.18571429 0.2 0.21428571 0.22857143 0.24285714 0.25714286 0.27142857 0.28571429 0.3 0.31428571 0.32857143 0.34285714 0.35714286 0.37142857 0.38571429 0.4 0.41428571 0.42857143 0.44285714 0.45714286 0.47142857 0.48571429 0.5 0.51428571 0.52857143 0.54285714 0.55714286 0.57142857 0.58571429 0.6 0.61428571 0.62857143 0.64285714 0.65714286 0.67142857 0.68571429 0.7 0.71428571 0.72857143 0.74285714 0.75714286 0.77142857 0.78571429 0.8 0.81428571 0.82857143 0.84285714 0.85714286 0.87142857 0.88571429 0.9 0.91428571 0.92857143 0.94285714 0.95714286 0.97142857 0.98571429 1 1 1 1 1 1
  line L11 (1.8967, 0.021) -> (1.6934, 0.557)
  arc A24 (2.0061, 1.416) -> (1.6934, 0.557) centre (2.348, 0.8052) ccw
  arc A25 (2.0061, 1.416) -> (2.1008, 1.4707) centre (0, 5) ccw
  arc A26 (3.001, 1.3119) -> (2.1008, 1.4707) centre (2.4588, 0.8692) ccw
  line L12 (3.001, 1.3119) -> (3.3636, 0.8679)
  spline S12 degree 5 poles (3.3636, 0.8679) (3.3666, 0.8642) (3.3727, 0.857) (3.3823, 0.8464) (3.3957, 0.833) (3.4135, 0.8172) (3.4319, 0.802) (3.4508, 0.7871) (3.47, 0.7725) (3.4893, 0.758) (3.5088, 0.7437) (3.5285, 0.7296) (3.5486, 0.7158) (3.5689, 0.7023) (3.5896, 0.6892) (3.6106, 0.6763) (3.6319, 0.6638) (3.6534, 0.6514) (3.6751, 0.6393) (3.697, 0.6273) (3.7191, 0.6156) (3.7413, 0.6041) (3.7638, 0.5927) (3.7865, 0.5817) (3.8094, 0.5708) (3.8324, 0.5602) (3.8557, 0.5497) (3.8791, 0.5395) (3.9027, 0.5295) (3.9265, 0.5197) (3.9504, 0.51) (3.9745, 0.5006) (3.9987, 0.4914) (4.0231, 0.4823) (4.0476, 0.4735) (4.0724, 0.4649) (4.0972, 0.4564) (4.1222, 0.4482) (4.1473, 0.4401) (4.1726, 0.4322) (4.198, 0.4246) (4.2236, 0.4171) (4.2493, 0.4098) (4.2751, 0.4027) (4.301, 0.3958) (4.3271, 0.3891) (4.3533, 0.3825) (4.3796, 0.3762) (4.4061, 0.37) (4.4326, 0.364) (4.4593, 0.3583) (4.4861, 0.3527) (4.513, 0.3473) (4.54, 0.342) (4.5671, 0.337) (4.5944, 0.3321) (4.6217, 0.3275) (4.6491, 0.323) (4.6767, 0.3187) (4.7043, 0.3146) (4.7321, 0.3107) (4.7599, 0.3069) (4.7879, 0.3034) (4.8159, 0.3) (4.844, 0.2968) (4.8723, 0.2938) (4.9006, 0.291) (4.929, 0.2884) (4.9575, 0.2859) (4.986, 0.2837) (5.0147, 0.2816) (5.0377, 0.2801) (5.055, 0.279) (5.0665, 0.2784) (5.0723, 0.2781) knots 0 0 0 0 0 0 0.01428571 0.02857143 0.04285714 0.05714286 0.07142857 0.08571429 0.1 0.11428571 0.12857143 0.14285714 0.15714286 0.17142857 0.18571429 0.2 0.21428571 0.22857143 0.24285714 0.25714286 0.27142857 0.28571429 0.3 0.31428571 0.32857143 0.34285714 0.35714286 0.37142857 0.38571429 0.4 0.41428571 0.42857143 0.44285714 0.45714286 0.47142857 0.48571429 0.5 0.51428571 0.52857143 0.54285714 0.55714286 0.57142857 0.58571429 0.6 0.61428571 0.62857143 0.64285714 0.65714286 0.67142857 0.68571429 0.7 0.71428571 0.72857143 0.74285714 0.75714286 0.77142857 0.78571429 0.8 0.81428571 0.82857143 0.84285714 0.85714286 0.87142857 0.88571429 0.9 0.91428571 0.92857143 0.94285714 0.95714286 0.97142857 0.98571429 1 1 1 1 1 1
  arc A27 (5.0723, 0.2781) -> (5.531, 0.8247) centre (0, 5) ccw
  spline S13 degree 5 poles (4.6534, 2.405) (4.6576, 2.4027) (4.6658, 2.3979) (4.6778, 2.3904) (4.6933, 2.3794) (4.712, 2.3647) (4.7302, 2.3492) (4.7481, 2.3332) (4.7658, 2.3168) (4.7834, 2.3003) (4.8009, 2.2836) (4.8182, 2.2666) (4.8353, 2.2493) (4.8521, 2.2316) (4.8687, 2.2135) (4.885, 2.195) (4.901, 2.1762) (4.9169, 2.1572) (4.9327, 2.1379) (4.9482, 2.1185) (4.9636, 2.0988) (4.9788, 2.0788) (4.9939, 2.0587) (5.0087, 2.0383) (5.0234, 2.0176) (5.0379, 1.9968) (5.0522, 1.9757) (5.0663, 1.9544) (5.0803, 1.9329) (5.0941, 1.9112) (5.1077, 1.8893) (5.1212, 1.8672) (5.1345, 1.845) (5.1476, 1.8225) (5.1606, 1.7999) (5.1734, 1.777) (5.186, 1.754) (5.1985, 1.7308) (5.2108, 1.7075) (5.2229, 1.6839) (5.2349, 1.6603) (5.2467, 1.6364) (5.2583, 1.6124) (5.2698, 1.5882) (5.2811, 1.5638) (5.2923, 1.5393) (5.3033, 1.5146) (5.3141, 1.4898) (5.3247, 1.4649) (5.3352, 1.4397) (5.3456, 1.4145) (5.3557, 1.3891) (5.3657, 1.3635) (5.3756, 1.3378) (5.3852, 1.312) (5.3947, 1.286) (5.4041, 1.2599) (5.4133, 1.2336) (5.4223, 1.2073) (5.4311, 1.1808) (5.4398, 1.1541) (5.4483, 1.1273) (5.4567, 1.1004) (5.4649, 1.0734) (5.4729, 1.0463) (5.4807, 1.019) (5.4884, 0.9916) (5.4959, 0.9641) (5.5033, 0.9364) (5.5105, 0.9087) (5.5175, 0.8808) (5.523, 0.8585) (5.527, 0.8416) (5.5297, 0.8304) (5.531, 0.8247) knots 0 0 0 0 0 0 0.01428571 0.02857143 0.04285714 0.05714286 0.07142857 0.08571429 0.1 0.11428571 0.12857143 0.14285714 0.15714286 0.17142857 0.18571429 0.2 0.21428571 0.22857143 0.24285714 0.25714286 0.27142857 0.28571429 0.3 0.31428571 0.32857143 0.34285714 0.35714286 0.37142857 0.38571429 0.4 0.41428571 0.42857143 0.44285714 0.45714286 0.47142857 0.48571429 0.5 0.51428571 0.52857143 0.54285714 0.55714286 0.57142857 0.58571429 0.6 0.61428571 0.62857143 0.64285714 0.65714286 0.67142857 0.68571429 0.7 0.71428571 0.72857143 0.74285714 0.75714286 0.77142857 0.78571429 0.8 0.81428571 0.82857143 0.84285714 0.85714286 0.87142857 0.88571429 0.9 0.91428571 0.92857143 0.94285714 0.95714286 0.97142857 0.98571429 1 1 1 1 1 1
  line L13 (4.6534, 2.405) -> (4.1532, 2.685)
  arc A28 (3.8405, 3.544) -> (4.1532, 2.685) centre (4.495, 3.2958) ccw
  arc A29 (3.8405, 3.544) -> (3.8779, 3.6468) centre (0, 5) ccw
  arc A30 (4.6696, 4.1038) -> (3.8779, 3.6468) centre (4.5388, 3.4161) ccw
  line L14 (4.6696, 4.1038) -> (5.2327, 3.9967)
  spline S14 degree 5 poles (5.2327, 3.9967) (5.2374, 3.9958) (5.2468, 3.9942) (5.2609, 3.9923) (5.2798, 3.9907) (5.3035, 3.9899) (5.3275, 3.9901) (5.3515, 3.9909) (5.3755, 3.992) (5.3996, 3.9933) (5.4238, 3.9949) (5.448, 3.9968) (5.4722, 3.9991) (5.4964, 4.0019) (5.5208, 4.0051) (5.5451, 4.0088) (5.5695, 4.0128) (5.5939, 4.0172) (5.6183, 4.0218) (5.6428, 4.0267) (5.6672, 4.0319) (5.6917, 4.0374) (5.7162, 4.0432) (5.7407, 4.0493) (5.7652, 4.0556) (5.7897, 4.0623) (5.8142, 4.0693) (5.8387, 4.0765) (5.8632, 4.084) (5.8877, 4.0917) (5.9123, 4.0997) (5.9368, 4.108) (5.9613, 4.1165) (5.9858, 4.1253) (6.0103, 4.1343) (6.0347, 4.1435) (6.0592, 4.153) (6.0837, 4.1628) (6.1081, 4.1728) (6.1325, 4.183) (6.1569, 4.1935) (6.1813, 4.2042) (6.2057, 4.2151) (6.23, 4.2262) (6.2543, 4.2376) (6.2786, 4.2492) (6.3029, 4.2611) (6.3271, 4.2731) (6.3513, 4.2854) (6.3755, 4.2979) (6.3997, 4.3106) (6.4238, 4.3235) (6.4479, 4.3367) (6.4719, 4.35) (6.4959, 4.3636) (6.5199, 4.3774) (6.5439, 4.3914) (6.5678, 4.4056) (6.5916, 4.42) (6.6154, 4.4347) (6.6392, 4.4495) (6.663, 4.4645) (6.6866, 4.4798) (6.7103, 4.4952) (6.7339, 4.5108) (6.7574, 4.5267) (6.7809, 4.5427) (6.8044, 4.559) (6.8278, 4.5754) (6.8511, 4.592) (6.8744, 4.6089) (6.893, 4.6225) (6.9069, 4.6328) (6.9162, 4.6397) (6.9208, 4.6432) knots 0 0 0 0 0 0 0.01428571 0.02857143 0.04285714 0.05714286 0.07142857 0.08571429 0.1 0.11428571 0.12857143 0.14285714 0.15714286 0.17142857 0.18571429 0.2 0.21428571 0.22857143 0.24285714 0.25714286 0.27142857 0.28571429 0.3 0.31428571 0.32857143 0.34285714 0.35714286 0.37142857 0.38571429 0.4 0.41428571 0.42857143 0.44285714 0.45714286 0.47142857 0.48571429 0.5 0.51428571 0.52857143 0.54285714 0.55714286 0.57142857 0.58571429 0.6 0.61428571 0.62857143 0.64285714 0.65714286 0.67142857 0.68571429 0.7 0.71428571 0.72857143 0.74285714 0.75714286 0.77142857 0.78571429 0.8 0.81428571 0.82857143 0.84285714 0.85714286 0.87142857 0.88571429 0.9 0.91428571 0.92857143 0.94285714 0.95714286 0.97142857 0.98571429 1 1 1 1 1 1
  arc A31 (6.9208, 4.6432) -> (6.9208, 5.3568) centre (0, 5) ccw
  spline S15 degree 5 poles (5.2327, 6.0033) (5.2374, 6.0042) (5.2468, 6.0058) (5.2609, 6.0077) (5.2798, 6.0093) (5.3035, 6.0101) (5.3275, 6.0099) (5.3515, 6.0091) (5.3755, 6.008) (5.3996, 6.0067) (5.4238, 6.0051) (5.448, 6.0032) (5.4722, 6.0009) (5.4964, 5.9981) (5.5208, 5.9949) (5.5451, 5.9912) (5.5695, 5.9872) (5.5939, 5.9828) (5.6183, 5.9782) (5.6428, 5.9733) (5.6672, 5.9681) (5.6917, 5.9626) (5.7162, 5.9568) (5.7407, 5.9507) (5.7652, 5.9444) (5.7897, 5.9377) (5.8142, 5.9307) (5.8387, 5.9235) (5.8632, 5.916) (5.8877, 5.9083) (5.9123, 5.9003) (5.9368, 5.892) (5.9613, 5.8835) (5.9858, 5.8747) (6.0103, 5.8657) (6.0347, 5.8565) (6.0592, 5.847) (6.0837, 5.8372) (6.1081, 5.8272) (6.1325, 5.817) (6.1569, 5.8065) (6.1813, 5.7958) (6.2057, 5.7849) (6.23, 5.7738) (6.2543, 5.7624) (6.2786, 5.7508) (6.3029, 5.7389) (6.3271, 5.7269) (6.3513, 5.7146) (6.3755, 5.7021) (6.3997, 5.6894) (6.4238, 5.6765) (6.4479, 5.6633) (6.4719, 5.65) (6.4959, 5.6364) (6.5199, 5.6226) (6.5439, 5.6086) (6.5678, 5.5944) (6.5916, 5.58) (6.6154, 5.5653) (6.6392, 5.5505) (6.663, 5.5355) (6.6866, 5.5202) (6.7103, 5.5048) (6.7339, 5.4892) (6.7574, 5.4733) (6.7809, 5.4573) (6.8044, 5.441) (6.8278, 5.4246) (6.8511, 5.408) (6.8744, 5.3911) (6.893, 5.3775) (6.9069, 5.3672) (6.9162, 5.3603) (6.9208, 5.3568) knots 0 0 0 0 0 0 0.01428571 0.02857143 0.04285714 0.05714286 0.07142857 0.08571429 0.1 0.11428571 0.12857143 0.14285714 0.15714286 0.17142857 0.18571429 0.2 0.21428571 0.22857143 0.24285714 0.25714286 0.27142857 0.28571429 0.3 0.31428571 0.32857143 0.34285714 0.35714286 0.37142857 0.38571429 0.4 0.41428571 0.42857143 0.44285714 0.45714286 0.47142857 0.48571429 0.5 0.51428571 0.52857143 0.54285714 0.55714286 0.57142857 0.58571429 0.6 0.61428571 0.62857143 0.64285714 0.65714286 0.67142857 0.68571429 0.7 0.71428571 0.72857143 0.74285714 0.75714286 0.77142857 0.78571429 0.8 0.81428571 0.82857143 0.84285714 0.85714286 0.87142857 0.88571429 0.9 0.91428571 0.92857143 0.94285714 0.95714286 0.97142857 0.98571429 1 1 1 1 1 1
  line L15 (5.2327, 6.0033) -> (4.6696, 5.8962)
  arc A32 (3.8779, 6.3532) -> (4.6696, 5.8962) centre (4.5388, 6.5839) ccw
  arc A33 (3.8779, 6.3532) -> (3.8405, 6.456) centre (0, 5) ccw
  arc A34 (4.1532, 7.315) -> (3.8405, 6.456) centre (4.495, 6.7042) ccw
  line L16 (4.1532, 7.315) -> (4.6534, 7.595)
  spline S16 degree 5 poles (4.6534, 7.595) (4.6576, 7.5973) (4.6658, 7.6021) (4.6778, 7.6096) (4.6933, 7.6206) (4.712, 7.6353) (4.7302, 7.6508) (4.7481, 7.6668) (4.7658, 7.6832) (4.7834, 7.6997) (4.8009, 7.7164) (4.8182, 7.7334) (4.8353, 7.7507) (4.8521, 7.7684) (4.8687, 7.7865) (4.885, 7.805) (4.901, 7.8238) (4.9169, 7.8428) (4.9327, 7.8621) (4.9482, 7.8815) (4.9636, 7.9012) (4.9788, 7.9212) (4.9939, 7.9413) (5.0087, 7.9617) (5.0234, 7.9824) (5.0379, 8.0032) (5.0522, 8.0243) (5.0663, 8.0456) (5.0803, 8.0671) (5.0941, 8.0888) (5.1077, 8.1107) (5.1212, 8.1328) (5.1345, 8.155) (5.1476, 8.1775) (5.1606, 8.2001) (5.1734, 8.223) (5.186, 8.246) (5.1985, 8.2692) (5.2108, 8.2925) (5.2229, 8.3161) (5.2349, 8.3397) (5.2467, 8.3636) (5.2583, 8.3876) (5.2698, 8.4118) (5.2811, 8.4362) (5.2923, 8.4607) (5.3033, 8.4854) (5.3141, 8.5102) (5.3247, 8.5351) (5.3352, 8.5603) (5.3456, 8.5855) (5.3557, 8.6109) (5.3657, 8.6365) (5.3756, 8.6622) (5.3852, 8.688) (5.3947, 8.714) (5.4041, 8.7401) (5.4133, 8.7664) (5.4223, 8.7927) (5.4311, 8.8192) (5.4398, 8.8459) (5.4483, 8.8727) (5.4567, 8.8996) (5.4649, 8.9266) (5.4729, 8.9537) (5.4807, 8.981) (5.4884, 9.0084) (5.4959, 9.0359) (5.5033, 9.0636) (5.5105, 9.0913) (5.5175, 9.1192) (5.523, 9.1415) (5.527, 9.1584) (5.5297, 9.1696) (5.531, 9.1753) knots 0 0 0 0 0 0 0.01428571 0.02857143 0.04285714 0.05714286 0.07142857 0.08571429 0.1 0.11428571 0.12857143 0.14285714 0.15714286 0.17142857 0.18571429 0.2 0.21428571 0.22857143 0.24285714 0.25714286 0.27142857 0.28571429 0.3 0.31428571 0.32857143 0.34285714 0.35714286 0.37142857 0.38571429 0.4 0.41428571 0.42857143 0.44285714 0.45714286 0.47142857 0.48571429 0.5 0.51428571 0.52857143 0.54285714 0.55714286 0.57142857 0.58571429 0.6 0.61428571 0.62857143 0.64285714 0.65714286 0.67142857 0.68571429 0.7 0.71428571 0.72857143 0.74285714 0.75714286 0.77142857 0.78571429 0.8 0.81428571 0.82857143 0.84285714 0.85714286 0.87142857 0.88571429 0.9 0.91428571 0.92857143 0.94285714 0.95714286 0.97142857 0.98571429 1 1 1 1 1 1
  arc A35 (5.531, 9.1753) -> (5.0723, 9.7219) centre (0, 5) ccw
  spline S17 degree 5 poles (3.3636, 9.1321) (3.3666, 9.1358) (3.3727, 9.143) (3.3823, 9.1536) (3.3957, 9.167) (3.4135, 9.1828) (3.4319, 9.198) (3.4508, 9.2129) (3.47, 9.2275) (3.4893, 9.242) (3.5088, 9.2563) (3.5285, 9.2704) (3.5486, 9.2842) (3.5689, 9.2977) (3.5896, 9.3108) (3.6106, 9.3237) (3.6319, 9.3362) (3.6534, 9.3486) (3.6751, 9.3607) (3.697, 9.3727) (3.7191, 9.3844) (3.7413, 9.3959) (3.7638, 9.4073) (3.7865, 9.4183) (3.8094, 9.4292) (3.8324, 9.4398) (3.8557, 9.4503) (3.8791, 9.4605) (3.9027, 9.4705) (3.9265, 9.4803) (3.9504, 9.49) (3.9745, 9.4994) (3.9987, 9.5086) (4.0231, 9.5177) (4.0476, 9.5265) (4.0724, 9.5351) (4.0972, 9.5436) (4.1222, 9.5518) (4.1473, 9.5599) (4.1726, 9.5678) (4.198, 9.5754) (4.2236, 9.5829) (4.2493, 9.5902) (4.2751, 9.5973) (4.301, 9.6042) (4.3271, 9.6109) (4.3533, 9.6175) (4.3796, 9.6238) (4.4061, 9.63) (4.4326, 9.636) (4.4593, 9.6417) (4.4861, 9.6473) (4.513, 9.6527) (4.54, 9.658) (4.5671, 9.663) (4.5944, 9.6679) (4.6217, 9.6725) (4.6491, 9.677) (4.6767, 9.6813) (4.7043, 9.6854) (4.7321, 9.6893) (4.7599, 9.6931) (4.7879, 9.6966) (4.8159, 9.7) (4.844, 9.7032) (4.8723, 9.7062) (4.9006, 9.709) (4.929, 9.7116) (4.9575, 9.7141) (4.986, 9.7163) (5.0147, 9.7184) (5.0377, 9.7199) (5.055, 9.721) (5.0665, 9.7216) (5.0723, 9.7219) knots 0 0 0 0 0 0 0.01428571 0.02857143 0.04285714 0.05714286 0.07142857 0.08571429 0.1 0.11428571 0.12857143 0.14285714 0.15714286 0.17142857 0.18571429 0.2 0.21428571 0.22857143 0.24285714 0.25714286 0.27142857 0.28571429 0.3 0.31428571 0.32857143 0.34285714 0.35714286 0.37142857 0.38571429 0.4 0.41428571 0.42857143 0.44285714 0.45714286 0.47142857 0.48571429 0.5 0.51428571 0.52857143 0.54285714 0.55714286 0.57142857 0.58571429 0.6 0.61428571 0.62857143 0.64285714 0.65714286 0.67142857 0.68571429 0.7 0.71428571 0.72857143 0.74285714 0.75714286 0.77142857 0.78571429 0.8 0.81428571 0.82857143 0.84285714 0.85714286 0.87142857 0.88571429 0.9 0.91428571 0.92857143 0.94285714 0.95714286 0.97142857 0.98571429 1 1 1 1 1 1
  line L17 (3.3636, 9.1321) -> (3.001, 8.6881)
  arc A36 (2.1008, 8.5293) -> (3.001, 8.6881) centre (2.4588, 9.1308) ccw
  arc A37 (2.1008, 8.5293) -> (2.0061, 8.584) centre (0, 5) ccw
  circle A38 centre (0, 5) radius 8.75
  circle A39 centre (0, 5) radius 7
  line L18 (2.8, 6.6166) -> (0, 8.2332)
  line L19 (0, 8.2332) -> (-2.8, 6.6166)
  line L20 (-2.8, 6.6166) -> (-2.8, 3.3834)
  line L21 (-2.8, 3.3834) -> (0, 1.7668)
  line L22 (0, 1.7668) -> (2.8, 3.3834)
  line L23 (2.8, 3.3834) -> (2.8, 6.6166)
  line L24 (1.75, 0, -1) -> (22.5, 0, -1)
  circle A40 centre (0, 5) radius 4.9
  circle A41 centre (0, 5) radius 1.75
  spline S18 degree 3 poles (-3.5989, 8.9321) (-3.7213, 9.0741) (-3.7554, 9.2013) (-3.8019, 9.3389) (-3.9533, 9.7872) (-3.9815, 10.303) (-3.9184, 10.8329) (-3.9156, 10.8561) (-3.9129, 10.8792) (-3.9101, 10.9023) knots 0 0 0 0 0.234809 0.234809 0.234809 1 1 1 1.034527 1.034527 1.034527 1.034527
  arc A42 (-3.1565, 11.3374) -> (-3.9101, 10.9023) centre (0, 5) ccw
  spline S19 degree 3 poles (-1.6059, 10.0827) (-1.6676, 10.2598) (-1.7607, 10.3529) (-1.8566, 10.4619) (-2.1692, 10.8173) (-2.6017, 11.0996) (-3.0923, 11.3099) (-3.1137, 11.3191) (-3.1351, 11.3282) (-3.1565, 11.3374) knots 0 0 0 0 0.234809 0.234809 0.234809 1 1 1 1.034527 1.034527 1.034527 1.034527
  line L25 (-1.417, 9.5415) -> (-1.6059, 10.0827)
  arc A43 (-1.417, 9.5415) -> (-0.795, 9.1823) centre (-0.8977, 9.7226) ccw
  arc A44 (-0.6834, 9.202) -> (-0.795, 9.1823) centre (0, 5) ccw
  arc A45 (-0.6834, 9.202) -> (-0.2217, 9.7522) centre (-0.7717, 9.7449) ccw
  line L26 (-0.2294, 10.3255) -> (-0.2217, 9.7522)
  spline S20 degree 3 poles (-0.2294, 10.3255) (-0.2319, 10.513) (-0.1763, 10.6323) (-0.1234, 10.7675) (0.0488, 11.2084) (0.3586, 11.6216) (0.7477, 11.987) (0.7647, 12.0029) (0.7817, 12.0189) (0.7986, 12.0348) knots 0 0 0 0 0.234809 0.234809 0.234809 1 1 1 1.034527 1.034527 1.034527 1.034527
  arc A46 (1.6556, 11.8837) -> (0.7986, 12.0348) centre (0, 5) ccw
  spline S21 degree 3 poles (2.037, 9.9258) (2.1035, 10.1012) (2.092, 10.2323) (2.0886, 10.3775) (2.0775, 10.8506) (1.9277, 11.3449) (1.6871, 11.8213) (1.6766, 11.8421) (1.6661, 11.8629) (1.6556, 11.8837) knots 0 0 0 0 0.234809 0.234809 0.234809 1 1 1 1.034527 1.034527 1.034527 1.034527
  line L27 (1.8337, 9.3898) -> (2.037, 9.9258)
  arc A47 (1.8337, 9.3898) -> (2.0793, 8.7149) centre (2.348, 9.1948) ccw
  arc A48 (2.1775, 8.6582) -> (2.0793, 8.7149) centre (0, 5) ccw
  arc A49 (2.1775, 8.6582) -> (2.8848, 8.7829) centre (2.4588, 9.1308) ccw
  line L28 (3.2474, 9.227) -> (2.8848, 8.7829)
  spline S22 degree 3 poles (3.2474, 9.227) (3.366, 9.3722) (3.4853, 9.4279) (3.6128, 9.4975) (4.028, 9.7245) (4.531, 9.8419) (5.0639, 9.8717) (5.0872, 9.873) (5.1104, 9.8743) (5.1337, 9.8756) knots 0 0 0 0 0.234809 0.234809 0.234809 1 1 1 1.034527 1.034527 1.034527 1.034527